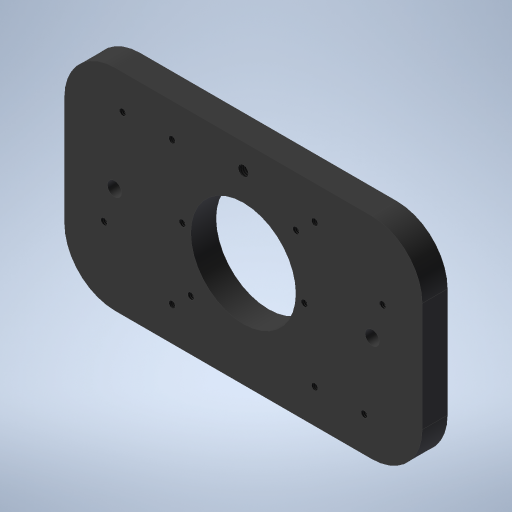
# Autodesk Inventor part: new-adapter-plate
Saved by Autodesk Inventor 2024 (Build 280153000, 153)
## iProperties
Created: 2023-09-14
Part Number: new-adapter-plate
Material: Generic
Document SubType Name: Modeling
Designer: raad
Density: 1 g/cm^3
Appearance: Default
Author: raad
Autodesk Inventor part; units mm, degrees
ref_plane "YZ Plane" through (0, 0, 0) normal (1, 0, 0) x (0, 1, 0)
ref_plane "XZ Plane" through (0, 0, 0) normal (0, 1, 0) x (-1, 0, 0)
ref_plane "XY Plane" through (0, 0, 0) normal (0, 0, 1) x (1, 0, 0)
sketch "Sketch1" plane through (0, 0, 0) normal (0, 0, 1) x (1, 0, 0)
  line L0 (-30.5, -25) -> (30.5, -25)
  line L1 (42.5, -13) -> (42.5, 13)
  line L2 (30.5, 25) -> (-30.5, 25)
  line L3 (-42.5, 13) -> (-42.5, -13)
  line L4 (-42.5, -25) -> (42.5, 25) construction
  line L5 (42.5, -25) -> (-42.5, 25) construction
  arc A0 (-30.5, 25) -> (-42.5, 13) centre (-30.5, 13) ccw
  arc A1 (-42.5, -13) -> (-30.5, -25) centre (-30.5, -13) ccw
  arc A2 (30.5, -25) -> (42.5, -13) centre (30.5, -13) ccw
  arc A3 (42.5, 13) -> (30.5, 25) centre (30.5, 13) ccw
  line L6 (-19.05, -19.05) -> (19.05, -19.05)
  line L7 (19.05, -19.05) -> (19.05, 19.05)
  line L8 (19.05, 19.05) -> (-19.05, 19.05)
  line L9 (-19.05, 19.05) -> (-19.05, -19.05)
  line L10 (-19.05, -19.05) -> (19.05, 19.05) construction
  line L11 (19.05, -19.05) -> (-19.05, 19.05) construction
  circle A4 centre (0, 0) radius 12.5
  line L12 (-19.05, 19.05) -> (-16.95, 19.05)
  line L13 (-16.95, 19.05) -> (-16.95, 16.95)
  circle A5 centre (-16.95, 16.95) radius 2.25
  line L14 (19.05, 19.05) -> (16.95, 19.05)
  line L15 (16.95, 19.05) -> (16.95, 16.95)
  line L16 (-19.05, -19.05) -> (-16.95, -19.05)
  line L17 (-16.95, -19.05) -> (-16.95, -16.95)
  line L18 (19.05, -19.05) -> (16.95, -19.05)
  line L19 (16.95, -19.05) -> (16.95, -16.95)
  circle A6 centre (16.95, 16.95) radius 2.25
  circle A7 centre (-16.95, -16.95) radius 2.25
  circle A8 centre (16.95, -16.95) radius 2.25
  line L20 (0, 0) -> (30.625, 0)
  line L21 (0, 0) -> (-30.625, 0)
  circle A9 centre (-30.625, 0) radius 3.2
  circle A10 centre (30.625, 0) radius 3.2
  circle A11 centre (0, 19.05) radius 2.85
  dimension "d0" = 85
  dimension "d1" = 50
  dimension "d2" = 12
  dimension "d3" = 38.1
  dimension "d4" = 38.1
  dimension "d5" = 25
  dimension "d6" = 2.1
  dimension "d7" = 2.1
  dimension "d8" = 4.5
  dimension "d9" = 2.1
  dimension "d10" = 2.1
  dimension "d11" = 2.1
  dimension "d12" = 2.1
  dimension "d13" = 2.1
  dimension "d14" = 2.1
  dimension "d15" = 4.5
  dimension "d16" = 4.5
  dimension "d17" = 4.5
  dimension "d18" = 30.625
  dimension "d19" = 30.625
  dimension "d20" = 6.4
  dimension "d21" = 6.4
  dimension "d22" = 5.7
  constraints: 44 end point, 17 point on line, 12 centre point, 8 point on circle, 8 tangent, 7 coincident, 5 midpoint, 4 parallel, 3 equal radius, 3 horizontal, 2 perpendicular
  measures "d0" distance of L5.end L4.end
  measures "d1" distance of L4.end L5.start
  measures "d2" radius of A0
  measures "d3" distance of L8.end L7.end
  measures "d4" distance of L7.end L6.end
  measures "d5" diameter of A4
  measures "d6" distance of L8.end L12.end
  measures "d7" distance of L12.end L13.end
  measures "d8" diameter of A5
  measures "d9" distance of L7.end L14.end
  measures "d10" distance of L14.end L15.end
  measures "d11" distance of L6.start L16.end
  measures "d12" distance of L16.end L17.end
  measures "d13" distance of L6.end L18.end
  measures "d14" distance of L18.end L19.end
  measures "d15" diameter of A6
  measures "d16" diameter of A7
  measures "d17" diameter of A8
  measures "d18" distance of L20.start L20.end
  measures "d19" distance of L20.start L21.end
  measures "d20" diameter of A9
  measures "d21" diameter of A10
  measures "d22" diameter of A11
extrude "Extrusion1" add sketch "Sketch1" against normal blind 6 contours A1 L3 A0 L2 A3 L1 A2 L0 | L9 A7 L6 | A9 | A10 | A7 L9 L6 | L6 A7 | A7 L9 | A7 L9 L21 A4 L20 L7 A8 L6 | A8 L7 L6 | L6 A8 | L9 A5 L8 A11 A6 L7 L20 A4 L21 | A8 L7 | A8 L7 L6 | A5 L9 | L9 A5 L8 | L21 L20 A4 | A4 L20 L21 | L9 L8 A5 | A6 L8 L7 | L7 A6 | A5 L8 | A6 L8 L7 | A6 L8 | A11 L8 | L8 A11
hole "Hole1" at (-30.625, 0, 0) at (30.625, 0, 0) direction (0, 0, -1) diameter 3.4 end through all clearance for "Flat Head Machine Screw" size "M3" standard "Ansi Metric M Profile"
hole "Hole2" at (0, 19.05, 0) direction (0, 0, -1) diameter 2.459 end through all thread size "M3x0.5" class "6H" standard "ISO Metric profile"
hole "Hole3" at (-16.95, 16.95, 0) at (16.95, 16.95, 0) at (16.95, -16.95, 0) at (-16.95, -16.95, 0) direction (0, 0, -1) diameter 1.567 end through all thread size "M2x0.4" class "6H" standard "ISO Metric profile"
hole "Hole4" at (0, 0, 0) direction (0, 0, -1) diameter 25 end through all
sketch "Sketch2" plane through (0, 0, -6) normal (0, 0, -1) x (-1, 0, 0)
  line L0 (42.5, 25) -> (14.5, 25)
  line L1 (14.5, 25) -> (14.5, 1)
  line L2 (42.5, 25) -> (42.5, 16.73)
  line L3 (42.5, 16.73) -> (28.7, 16.73)
  line L4 (-42.5, -25) -> (-42.5, -16.73)
  line L5 (-42.5, -16.73) -> (-28.7, -16.73)
  line L6 (-42.5, -25) -> (-14.5, -25)
  line L7 (30.5, -25) -> (-30.5, -25) projected
  line L8 (-14.5, -25) -> (-14.5, -1)
  line L9 (-42.5, 25) -> (-12.5, 25)
  line L10 (-12.5, 25) -> (-12.5, 13)
  line L11 (42.5, -25) -> (12.5, -25)
  line L12 (12.5, -25) -> (12.5, -13)
  line L13 (-42.5, 25) -> (-42.5, 8)
  line L14 (-42.5, 8) -> (-33.11, 8)
  line L15 (42.5, -25) -> (42.5, -8)
  line L16 (42.5, -8) -> (33.11, -8)
  point P0 (0, 0)
  dimension "d53" = 28
  dimension "d54" = 24
  dimension "d55" = 8.27
  dimension "d56" = 13.8
  dimension "d57" = 8.27
  dimension "d58" = 13.8
  dimension "d59" = 28
  dimension "d60" = 24
  dimension "d61" = 30
  dimension "d62" = 12
  dimension "d63" = 30
  dimension "d64" = 12
  dimension "d65" = 17
  dimension "d66" = 9.39
  dimension "d67" = 17
  dimension "d68" = 9.39
  constraints: 32 end point, 8 perpendicular, 4 vertical, 2 horizontal, 2 point on line
  measures "d53" distance of L0.start L0.end
  measures "d54" distance of L0.end L1.end
  measures "d55" distance of L0.start L2.end
  measures "d56" distance of L2.end L3.end
  measures "d57" distance of L4.start L4.end
  measures "d58" distance of L4.end L5.end
  measures "d59" distance of L4.start L6.end
  measures "d60" distance of L6.end L8.end
  measures "d61" distance of L9.start L9.end
  measures "d62" distance of L9.end L10.end
  measures "d63" distance of L11.start L11.end
  measures "d64" distance of L11.end L12.end
  measures "d65" distance of L9.start L13.end
  measures "d66" distance of L13.end L14.end
  measures "d67" distance of L11.start L15.end
  measures "d68" distance of L15.end L16.end
hole "Hole5" at (33.11, 8, -6) at (12.5, 13, -6) at (-28.7, 16.73, -6) at (-14.5, 1, -6) at (-33.11, -8, -6) at (-12.5, -13, -6) at (14.5, -1, -6) at (28.7, -16.73, -6) direction (0, 0, 1) diameter 1.567 end through all thread size "M2x0.4" class "6H" standard "ISO Metric profile"
body "Solid1"
